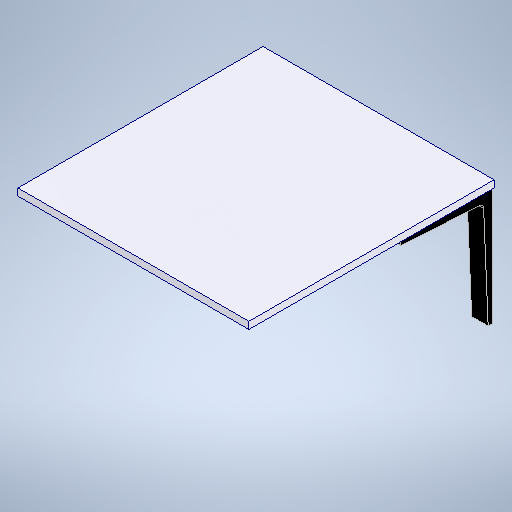
# Autodesk Inventor part: ShedDesk
Saved by Autodesk Inventor 2025 (Build 290162010, 162A)
## iProperties
Created: 2024-08-20
Part Number: ShedDesk
Material: Generic
Document SubType Name: Modeling
Designer: max_d
Density: 1 g/cm^3
Appearance: Default
Author: max_d
Autodesk Inventor part; units mm, degrees
ref_plane "YZ Plane" through (0, 0, 0) normal (1, 0, 0) x (0, 1, 0)
sketch "Sketch1" plane through (0, 0, 0) normal (0, 1, 0) x (-1, 0, 0)
  line L0 (245, 260) -> (-245, 260)
  line L1 (-245, 260) -> (-245, -260)
  line L2 (-245, -260) -> (245, -260)
  line L3 (245, -260) -> (245, 260)
  line L4 (245, 260) -> (-245, -260) construction
  line L5 (-245, 260) -> (245, -260) construction
  point P0 (0, 0)
  dimension "d0" = 490
  dimension "d1" = 520
  constraints: 12 end point, 2 midpoint, 2 parallel, 1 horizontal, 1 perpendicular
  measures "d0" distance of L2.end L1.end
  measures "d1" distance of L1.end L0.end
extrude "Extrusion1" add sketch "Sketch1" along normal blind 15
ref_plane "Work Plane1" through (242.5, 0, 260) normal (1, 0, 0) x (0, 0, -1)
sketch "Sketch2" plane through (242.5, 0, 260) normal (1, 0, 0) x (0, 0, -1)
  line L0 (0, 0) -> (520, 0) projected
  line L1 (520, 0) -> (520, -250)
  line L2 (520, -250) -> (510, -250)
  line L3 (510, -250) -> (500, -20)
  line L4 (500, -20) -> (325, -10)
  line L5 (325, -10) -> (325, 0)
  line L6 (520, 0) -> (325, 0)
  line L7 (500, -20) -> (500, 0) construction
  line L8 (500, -20) -> (520, -20) construction
  point P0 (260, 0)
  dimension "d5" = 10
  dimension "d6" = 20
  dimension "d7" = 195
  dimension "d8" = 250
  constraints: 16 end point, 5 perpendicular, 3 point on line, 2 vertical, 1 collinear
  measures "d5" distance of L1.end L2.end
  measures "d6" distance of L3.end L8.end
  measures "d7" distance between parallel lines of L1 L5
  measures "d8" distance between parallel lines of L2 L0
extrude "Extrusion2" add sketch "Sketch2" against normal blind 35 separate body
fillet "Fillet1" radius 10 1 edges at (225, -20, -240)
ref_plane "Work Plane2" through (0, 0, 260) normal (1, 0, 0) x (0, 0, -1)
mirror "Mirror1" about plane through (0, 0, 260) normal (1, 0, 0) of "Extrusion2" bodies 2
body "Solid1"
body "Solid2"
